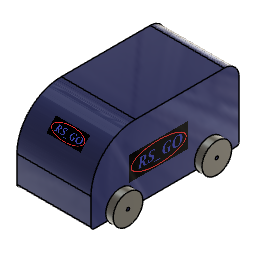
rs_go (Autodesk Fusion 360 design; units mm, degrees)
Autodesk Fusion 360 part; units mm, degrees
sketch "Sketch1" plane through (0, 0, 0) normal (1, 0, 0) x (0, 1, 0)
  line L0 (5, 15) -> (505, 15)
  line L1 (505, 15) -> (505, 265)
  line L2 (505, 265) -> (5, 265)
  line L3 (5, 265) -> (5, 15)
  dimension "d1" = 500
  dimension "d2" = 250
  constraint horizontal L0
  constraint vertical L1
  constraint horizontal L2
  constraint vertical L3
  measures "d1" distance of L0.start L0.end
  measures "d2" distance of L0.start L2.end
extrude "Extrude1" add sketch "Sketch1" along normal blind 250 makes body 1
sketch "Sketch2" plane through (250, 0, 0) normal (1, 0, 0) x (0, 1, 0)
  line L0 (5, 265) -> (5, 15)
  line L1 (5, 15) -> (505, 15)
  line L2 (505, 15) -> (505, 265)
  line L3 (505, 265) -> (5, 265)
  circle A0 centre (105, 40) radius 5
  dimension "d7" = 10
  measures "d7" diameter of A0
extrude "Extrude2" add sketch "Sketch2" along normal blind 25 contours A0 bodies 1
sketch "Sketch3" plane through (250, 0, 0) normal (1, 0, 0) x (0, 1, 0)
  circle A0 centre (105, 40) radius 5
  line L0 (5, 265) -> (5, 15)
  line L1 (5, 15) -> (505, 15)
  line L2 (505, 15) -> (505, 265)
  line L3 (505, 265) -> (5, 265)
  circle A1 centre (405, 40) radius 5
  dimension "d12" = 10
  measures "d12" diameter of A1
extrude "Extrude3" add sketch "Sketch3" along normal blind 25 contours A1 bodies 1
sketch "Sketch4" plane through (0, 0, 0) normal (-1, 0, 0) x (0, -1, 0)
  line L0 (-5, 15) -> (-5, 265)
  line L1 (-5, 265) -> (-505, 265)
  line L2 (-505, 265) -> (-505, 15)
  line L3 (-505, 15) -> (-5, 15)
  circle A0 centre (-405, 40) radius 5
  dimension "d17" = 10
  measures "d17" diameter of A0
extrude "Extrude4" add sketch "Sketch4" along normal blind 25 contours A0 bodies 1
sketch "Sketch5" plane through (0, 0, 0) normal (-1, 0, 0) x (0, -1, 0)
  circle A0 centre (-405, 40) radius 5
  line L0 (-5, 15) -> (-5, 265)
  line L1 (-5, 265) -> (-505, 265)
  line L2 (-505, 265) -> (-505, 15)
  line L3 (-505, 15) -> (-5, 15)
  circle A1 centre (-105, 40) radius 5
  dimension "d22" = 10
  measures "d22" diameter of A1
extrude "Extrude5" add sketch "Sketch5" along normal blind 25 contours A1 bodies 1
move_body "Move1" bodies 1 to x (1, 0, 0) y (0, 1, 0) z (0, 0, 1) at (0, 16.4616, 16.4616)
move_body "Move2" bodies 1 to x (1, 0, 0) y (0, 1, 0) z (0, 0, 1) at (-250, -21.4616, -31.4616)
move_body "Move3" bodies 1 to x (1, 0, 0) y (0, 1, 0) z (0, 0, 1) at (0, 0, 25)
copy_body "Body->Comp1" bodies 1 removing the originals makes body 2 in component "base_link"
fillet "Fillet1" radius 150 1 edges at (-125, 0, 275) on bodies 2 in component "base_link"
fillet "Fillet2" radius 50 1 edges at (-125, 500, 275) on bodies 2 in component "base_link"
fillet "Fillet3" radius 10 1 edges at (-125, 0, 25) on bodies 2 in component "base_link"
fillet "Fillet4" radius 10 1 edges at (-125, 500, 25) on bodies 2 in component "base_link"
sketch "Sketch7" plane through (0, 0, 0) normal (1, 0, 0) x (0, 1, 0)
  circle A0 centre (400, 50) radius 5
  circle A1 centre (100, 50) radius 5
  arc A2 (490, 25) -> (500, 35) centre (490, 35) ccw
  line L0 (500, 35) -> (500, 225)
  arc A3 (500, 225) -> (450, 275) centre (450, 225) ccw
  line L1 (450, 275) -> (150, 275)
  arc A4 (150, 275) -> (0, 125) centre (150, 125) ccw
  line L2 (0, 125) -> (0, 35)
  arc A5 (0, 35) -> (10, 25) centre (10, 35) ccw
  line L3 (10, 25) -> (490, 25)
  circle A6 centre (-180, 170) radius 50
  circle A7 centre (-180, 170) radius 5
  dimension "d39" = 100
  dimension "d40" = 10
  constraint concentric A6 A7
  measures "d39" diameter of A6
  measures "d40" diameter of A7
extrude "Extrude6" add sketch "Sketch7" along normal blind 25 separate body contours A6 makes body 3
copy_body "Body->Comp2" bodies 3 removing the originals makes body 4 in component "front_left_wheel"
sketch "Sketch8" plane through (0, 0, 0) normal (1, 0, 0) x (0, 1, 0)
  circle A0 centre (-398.2463, 233.6759) radius 50
  circle A1 centre (-398.2463, 233.6759) radius 5
  dimension "d47" = 100
  dimension "d48" = 10
  constraint concentric A0 A1
  measures "d47" diameter of A0
  measures "d48" diameter of A1
extrude "Extrude7" add sketch "Sketch8" along normal blind 25 separate body makes body 5
copy_body "Body->Comp3" bodies 5 removing the originals makes body 6 in component "back_left_wheel"
sketch "Sketch9" plane through (0, 0, 0) normal (1, 0, 0) x (0, 1, 0)
  circle A0 centre (-313.2933, 173.074) radius 50
  circle A1 centre (-313.2933, 173.074) radius 5
  dimension "d55" = 100
  dimension "d56" = 10
  constraint concentric A0 A1
  measures "d55" diameter of A0
  measures "d56" diameter of A1
extrude "Extrude8" add sketch "Sketch9" along normal blind 25 separate body makes body 7
copy_body "Body->Comp4" bodies 7 removing the originals makes body 8 in component "front_right_wheel"
sketch "Sketch10" plane through (0, 0, 0) normal (1, 0, 0) x (0, 1, 0)
  circle A0 centre (-338.4084, 168.2563) radius 50
  circle A1 centre (-338.4084, 168.2563) radius 5
  dimension "d63" = 100
  dimension "d64" = 10
  constraint concentric A0 A1
  measures "d63" diameter of A0
  measures "d64" diameter of A1
extrude "Extrude9" add sketch "Sketch10" along normal blind 25 separate body makes body 9
copy_body "Body->Comp5" bodies 9 removing the originals makes body 10 in component "back_right_wheel"
component "base_link" placed x (1, 0, 0) y (0, 1, 0) z (0, 0, 1) at (0, 0, 0)
component "front_left_wheel" placed x (1, 0, 0) y (0, 1, 0) z (0, 0, 1) at (0, 280, -120)
component "back_left_wheel" placed x (1, 0, 0) y (0, 1, 0) z (0, 0, 1) at (0, 798.2463, -183.6759)
component "front_right_wheel" placed x (1, 0, 0) y (0, 1, 0) z (0, 0, 1) at (-275, 413.2933, -123.074)
component "back_right_wheel" placed x (1, 0, 0) y (0, 1, 0) z (0, 0, 1) at (-275, 738.4084, -118.2563)
